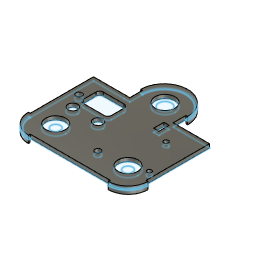
Carriage_Plate (Autodesk Fusion 360 design; units mm, degrees)
Autodesk Fusion 360 part; units mm, degrees
sketch "Back_Plate" plane through (0, 0, 0) normal (0, 0, 1) x (1, 0, 0)
  line L0 (-32.1, -22) -> (-32.1, 13)
  line L1 (12, 20) -> (12, 13)
  line L2 (12.1, 10.65) -> (9.2, 10.65)
  arc A0 (-22.1, -32) -> (-32.1, -22) centre (-22.1, -22) cw
  arc A1 (-24.1, -0.6) -> (-22.1, -2.6) centre (-22.1, -0.6) ccw
  line L3 (9.2, 10.65) -> (9.2, 5)
  line L4 (-22.1, -2.6) -> (-10.6, -2.6)
  arc A2 (32.1, -22) -> (22.1, -32) centre (22.1, -22) cw
  line L5 (32.1, 13) -> (32.1, -22)
  arc A3 (-12, 20) -> (12, 20) centre (0, 20) cw
  line L6 (12, 13) -> (15.1, 13)
  line L7 (22.1, -32) -> (-22.1, -32)
  line L8 (-12, 13) -> (-12, 20)
  line L9 (-15.1, 13) -> (-12, 13)
  line L10 (15.1, 13) -> (32.1, 13)
  line L11 (-8.6, -0.6) -> (-8.6, 6.4)
  arc A4 (-10.6, -2.6) -> (-8.6, -0.6) centre (-10.6, -0.6) ccw
  line L12 (12.1, 5) -> (12.1, 10.65)
  line L13 (-32.1, 13) -> (-15.1, 13)
  circle A5 centre (-23.35, -7.2) radius 2.65
  circle A6 centre (20, -20) radius 5.5
  arc A7 (22.1, -33) -> (33.1, -22) centre (22.1, -22) ccw
  arc A8 (12.1, 20) -> (-12.1, 20) centre (0, 20) ccw
  line L14 (-10.6, 8.4) -> (-22.1, 8.4)
  line L15 (-22.1, -33) -> (-22.1, -32)
  arc A9 (22.1, -32.1) -> (32.2, -22) centre (22.1, -22) ccw
  line L16 (-24.1, 6.4) -> (-24.1, -0.6)
  line L17 (13, 20) -> (12, 20)
  circle A10 centre (28.6, -16.8) radius 1.25
  circle A11 centre (-9.35, -7.2) radius 2.65
  circle A12 centre (0, 20.5) radius 3.5
  line L18 (33.1, -22) -> (32.1, -22)
  line L19 (9.2, 5) -> (12.1, 5)
  arc A13 (32.1, -22) -> (22.1, -32) centre (22.1, -22) cw
  arc A14 (-22.1, 8.4) -> (-24.1, 6.4) centre (-22.1, 6.4) ccw
  arc A15 (-33.1, -22) -> (-22.1, -33) centre (-22.1, -22) ccw
  circle A16 centre (19.1, 2) radius 1.25
  circle A17 centre (-20, -20) radius 5.5
  arc A18 (12, 20) -> (-12, 20) centre (0, 20) ccw
  arc A19 (-32.2, -22) -> (-22.1, -32.1) centre (-22.1, -22) ccw
  line L20 (-12, 20) -> (-13, 20)
  circle A20 centre (-20, -20) radius 2.5
  circle A21 centre (20, -20) radius 2.5
  line L21 (22.1, -32) -> (22.1, -33)
  circle A22 centre (-27.6, 0.5) radius 1.7
  circle A23 centre (4.6, -21.3) radius 1.6
  circle A24 centre (0, 20.5) radius 5.5
  line L22 (-32.1, -22) -> (-33.1, -22)
  arc A25 (-8.6, 6.4) -> (-10.6, 8.4) centre (-10.6, 6.4) ccw
  arc A26 (-22.1, -32) -> (-32.1, -22) centre (-22.1, -22) cw
  arc A27 (13, 20) -> (-13, 20) centre (0, 20) ccw
extrude "Extrude1" add sketch "Back_Plate" along normal blind 2 contours L0 L1 A0 A2 L5 A3 L6 L7 L8 L9 L10 L13 A13 A18 A26 | A0 L15 A19 L22 A26 | L15 A15 A19 L22 | A2 A9 L18 A13 L21 | A7 A9 L18 L21 | A3 A8 L17 A18 L20 | A8 L17 L20 A27
extrude "Extrude2" add sketch "Back_Plate" against normal blind 2 contours L15 A15 A19 L22 | A7 A9 L18 L21 | A8 L17 L20 A27
